Autodesk Inventor part; units mm, degrees
(part 2 of 2)
  spline S249 degree 2 poles (-24.2637, -25.4906) (-23.9967, -25.1794) (-23.3294, -24.8342) (-22.9607, -24.7991) knots 0 0 0 1 2 2 2
  spline S250 degree 2 poles (-22.9607, -24.7991) (-22.5781, -24.7629) (-21.8179, -25.0376) (-21.4543, -25.3497) knots 0 0 0 1 2 2 2
  spline S251 degree 2 poles (-21.4543, -25.3497) (-21.1056, -25.6489) (-20.5681, -26.4031) (-20.4354, -26.7188) knots 0 0 0 1 2 2 2
  line L266 (-20.4354, -26.7188) -> (-20.9984, -27.3748)
  line L267 (-20.9984, -27.3748) -> (-21.0434, -27.3362)
  spline S252 degree 2 poles (-21.0434, -27.3362) (-21.1161, -27.0265) (-21.5507, -26.1978) (-21.8768, -25.918) knots 0 0 0 1 2 2 2
  spline S253 degree 2 poles (-21.8768, -25.918) (-22.068, -25.7539) (-22.5534, -25.5457) (-22.7999, -25.575) knots 0 0 0 1 2 2 2
  spline S254 degree 2 poles (-22.7999, -25.575) (-23.0426, -25.6076) (-23.4569, -25.8249) (-23.6725, -26.0761) knots 0 0 0 1 2 2 2
  spline S255 degree 2 poles (-23.6725, -26.0761) (-23.888, -26.3272) (-24.0217, -26.7789) (-23.9709, -26.9852) knots 0 0 0 1 2 2 2
  spline S256 degree 2 poles (-23.9709, -26.9852) (-23.9201, -27.1915) (-23.6251, -27.5683) (-23.4152, -27.7485) knots 0 0 0 1 2 2 2
  line L268 (-23.4152, -27.7485) -> (-23.1527, -27.9737)
  line L269 (-23.1527, -27.9737) -> (-23.5935, -28.4873)
  line L270 (-23.5935, -28.4873) -> (-23.7997, -28.3104)
  spline S257 degree 2 poles (-23.7997, -28.3104) (-24.2158, -27.9533) (-25.0817, -27.9003) (-25.4066, -28.2789) knots 0 0 0 1 2 2 2
  spline S258 degree 2 poles (-25.4066, -28.2789) (-25.5578, -28.4551) (-25.6384, -28.8221) (-25.594, -28.9904) knots 0 0 0 1 2 2 2
  spline S259 degree 2 poles (-25.594, -28.9904) (-25.5453, -29.1688) (-25.3151, -29.477) (-25.1539, -29.6154) knots 0 0 0 1 2 2 2
  line L271 (-24.6099, -22.4939) -> (-23.9396, -23.2062)
  line L272 (-23.9396, -23.2062) -> (-24.7886, -24.0052)
  line L273 (-24.7886, -24.0052) -> (-25.4589, -23.2929)
  line L274 (-25.4589, -23.2929) -> (-24.6099, -22.4939)
  spline S260 degree 2 poles (-29.2327, -19.8276) (-28.8823, -19.5621) (-28.1138, -19.333) (-27.7381, -19.3707) knots 0 0 0 1 2 2 2
  spline S261 degree 2 poles (-27.7381, -19.3707) (-27.3625, -19.4083) (-26.6441, -19.8247) (-26.3577, -20.2026) knots 0 0 0 1 2 2 2
  spline S262 degree 2 poles (-26.3577, -20.2026) (-26.0951, -20.5491) (-25.7355, -21.3427) (-25.6696, -21.6832) knots 0 0 0 1 2 2 2
  line L275 (-25.6696, -21.6832) -> (-26.3586, -22.2054)
  line L276 (-26.3586, -22.2054) -> (-26.3944, -22.1581)
  spline S263 degree 2 poles (-26.3944, -22.1581) (-26.396, -22.0415) (-26.4661, -21.6546) (-26.5314, -21.4375) knots 0 0 0 1 2 2 2
  spline S264 degree 2 poles (-26.5314, -21.4375) (-26.6107, -21.1939) (-26.7775, -20.8183) (-26.9297, -20.6175) knots 0 0 0 1 2 2 2
  spline S265 degree 2 poles (-26.9297, -20.6175) (-27.0789, -20.4206) (-27.5011, -20.1579) (-27.7561, -20.1404) knots 0 0 0 1 2 2 2
  spline S266 degree 2 poles (-27.7561, -20.1404) (-27.9942, -20.1288) (-28.4756, -20.2952) (-28.7354, -20.4921) knots 0 0 0 1 2 2 2
  spline S267 degree 2 poles (-28.7354, -20.4921) (-28.9953, -20.689) (-29.2186, -21.0813) (-29.2274, -21.2988) knots 0 0 0 1 2 2 2
  spline S268 degree 2 poles (-29.2274, -21.2988) (-29.245, -21.5291) (-29.0371, -22.0161) (-28.8491, -22.2641) knots 0 0 0 1 2 2 2
  spline S269 degree 2 poles (-28.8491, -22.2641) (-28.6463, -22.5319) (-28.1608, -23.0008) (-28.003, -23.1353) knots 0 0 0 1 2 2 2
  line L277 (-28.003, -23.1353) -> (-30.5071, -25.0329)
  line L278 (-30.5071, -25.0329) -> (-32.527, -22.3674)
  line L279 (-32.527, -22.3674) -> (-31.9561, -21.9347)
  line L280 (-31.9561, -21.9347) -> (-30.4106, -23.9743)
  line L281 (-30.4106, -23.9743) -> (-29.1153, -22.9927)
  spline S270 degree 2 poles (-29.1153, -22.9927) (-29.2205, -22.8865) (-29.4054, -22.6671) (-29.477, -22.5726) knots 0 0 0 1 2 2 2
  spline S271 degree 2 poles (-29.477, -22.5726) (-29.7604, -22.1985) (-30.0292, -21.5902) (-30.0271, -21.2168) knots 0 0 0 1 2 2 2
  spline S272 degree 2 poles (-30.0271, -21.2168) (-30.028, -20.8393) (-29.6737, -20.1618) (-29.2327, -19.8276) knots 0 0 0 1 2 2 2
  dimension "d30" = 66.675
  constraints: 1 centre point, 1 coincident, 1 other
  measures "d30" diameter of A0
extrude "Extrusion4" cut sketch "Sketch5" against normal blind 1.27 contours L170 L171 L172 L173 | L178 L179 L180 L181 L182 L183 S191 L184 L185 L186 L187 | L188 L189 L190 L191 | L210 L199 L200 L201 L202 L203 L204 L205 L206 L207 L208 L209 | L259 L260 L261 L262 | L271 L272 L273 L274 | L29 L30 L31 L32 | L37 L38 L39 L40 | L48 L49 S38 S39 S40 S41 S42 S43 L50 L51 S44 S45 S46 S47 S48 L52 L53 | L97 L98 L99 L100 | L101 L102 S80 S81 S82 S83 S84 S85 L103 L104 S86 S87 S88 S89 S90 L105 L106 | L107 L108 L109 L110 | L111 L112 S91 S92 S93 S94 S95 S96 L113 L114 S97 S98 S99 S100 S101 L115 L116 | S147 S148 A0 | A0 S148 S149 S150 S147 | S165 S166 S167 S168 L152 S169 S170 S171 L153 L154 S172 S173 S174 L155 L156 L157 S163 S164 A0 | A0 S164 S165 | S139 S140 A0 | A0 S140 S141 S142 S139 | S131 S132 A0 | A0 S132 L128 L130 L131 L132 S133 S134 S131 | S194 L192 L193 S195 S196 S197 S198 S199 S200 S201 L194 L195 L196 L197 L198 S202 S203 S204 S192 S193 A0 | A0 S193 S194 | L128 L129 L130 A0 | S130 S115 A0 | A0 S115 L124 L125 S116 S117 S118 S119 S120 S121 S122 S123 L126 L127 S124 S125 S126 S127 S128 S129 S130 | S215 S216 S217 S218 L237 S219 S220 S221 L238 L239 S222 S223 S224 L240 L241 L242 S213 S214 A0 | A0 S214 S215 | S103 S104 A0 | A0 S104 L117 L118 S105 S106 S107 S108 S109 S110 S111 L119 L120 L121 L122 L123 S112 S113 S114 S102 S103 | S251 L266 L267 S252 S253 S254 S255 S256 L268 L269 L270 S257 S258 S259 S241 S242 L263 L264 S243 S244 S245 S246 L265 S247 S248 S249 S250 A0 | A0 S250 S251 | S262 L275 L276 S263 S264 S265 S266 S267 S268 S269 L277 L278 L279 L280 L281 S270 S271 S272 S260 S261 A0 | A0 S261 S262 | S79 S75 A0 | A0 S75 L80 L81 L82 L83 L84 L85 L86 L87 L88 L89 L90 S76 S77 S78 L91 L92 S79 | S0 S1 S2 S3 L12 L13 S4 S5 S6 L14 L15 S7 S8 A0 | A0 S8 S0 | S63 S64 A0 | A0 S64 L61 L62 S65 S66 S67 S68 S69 S70 S71 L63 L64 L65 L66 L67 S72 S73 S74 S62 S63 | S14 S15 S16 S13 A0 | A0 S13 S14 | S50 S51 A0 | A0 S51 L54 L55 S52 S53 S54 S55 S56 S57 S58 L56 L57 L58 L59 L60 S59 S60 S61 S49 S50 | S27 L41 L42 S28 S29 S30 S31 S32 S33 S34 L43 L44 L45 L46 L47 S35 S36 S37 S25 S26 A0 | A0 S26 S27 | L0 L1 L2 L3 L4 L5 L6 L7 L8 L9 L10 L11 | L17 L18 L19 L20 L21 L22 L23 L24 L25 L26 L27 L28 | L33 L34 L35 L36 | L68 L69 L70 L71 L72 L73 L74 L75 L76 L77 L78 L79 | L93 L94 L95 L96 | L134 L135 L136 L137 | S155 S156 L138 L139 L140 S157 S158 | L144 L145 L146 L147 | L148 L149 L150 L151 | L159 S179 S180 S181 S182 L160 L161 L162 S183 S184 S185 L163 L164 L165 L166 L167 S186 S187 S188 S189 S190 L168 L169 | L174 L175 L176 L177 | L211 L212 L213 L214 L215 L216 L217 L218 L219 L220 L221 L222 | S205 S206 L223 L224 L225 S207 S208 | L229 L230 L231 L232 | L233 L234 L235 L236 | L244 S229 S230 S231 S232 L245 L246 L247 S233 S234 S235 L248 L249 L250 L251 L252 S236 S237 S238 S239 S240 L253 L254 | L255 L256 L257 L258
chamfer "Chamfer3" distance 1.5875 angle 45 2 edges at (-17.096, 39.2076, 8.4042) (17.096, 14.4426, 8.4042)
equation "\"d0\" = spoolHeight"
equation "\"d1\" = supportChannels"
equation "\"d2\" = spoolInteriroRadius"
equation "\"d3\" = spoolExteriorRadius"
equation "\"d4\" = spoolFiletRadius"
equation "\"d5\" = spoolFiletRadius"
equation "\"d8\" = hexDiameter"
equation "\"d17\" = holeCenter"
equation "\"d18\" = holeCenter"
equation "\"d19\" = holeForString"
equation "\"d20\" = stringHoleCenterFromHexShaft"
equation "\"d21\" = stringHoleCenterFromHexShaft"
equation "\"d27\" = hexHoleChamfer"
equation "\"d30\" = textCircleDiameter"
equation "\"d31\" = textDepth"
equation "\"d33\" = stringHoleChamfer"
equation "\"holeForString\" = stringDiameter + clearanceForString"
equation "\"stringDiameter\" = 3"
equation "\"clearanceForString\" = 0.5"
equation "\"spoolHeight\" = 57.15"
equation "\"hexShaftDiameter\" = 12.7"
equation "\"clearanceForHexShaft\" = 0.5715"
equation "\"hexDiameter\" = hexShaftDiameter + clearanceForHexShaft"
equation "\"supportChannels\" = 7.62"
equation "\"spoolInteriorDiameter\" = 38.1"
equation "\"spoolInteriroRadius\" = 0.5 * spoolInteriorDiameter"
equation "\"spoolExteriorDiameter\" = 88.9"
equation "\"spoolExteriorRadius\" = 0.5 * spoolExteriorDiameter"
equation "\"spoolFiletRadius\" = 0.5 * supportChannels"
equation "\"holeCenter\" = 0.25 * spoolHeight - 0.75 * supportChannels"
equation "\"hexHoleChamfer\" = 1.5875"
equation "\"stringHoleCenterFromHexShaft\" = 0.5 * hexDiameter + 0.5 * holeForString"
equation "\"textCircleDiameter\" = 0.75 * spoolExteriorDiameter"
equation "\"textHeight\" = 6.096"
equation "\"textDepth\" = 1.27"
equation "\"stringHoleChamfer\" = 1.5875"
body "Solid1"
